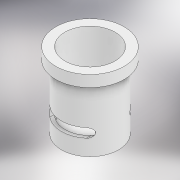
# Autodesk Inventor part: EndEffectorRotational
Saved by Autodesk Inventor 2020.3 (Build 243373000, 373)
## iProperties
Created: 2021-08-11
Part Number: EndEffectorRotational
Material: ABS Plastic
Document SubType Name: Modeling
Designer: justi
Density: 1.06 g/cm^3
Appearance: Smooth - White
Author: justi
Autodesk Inventor part; units mm, degrees
ref_plane "YZ Plane" through (0, 0, 0) normal (1, 0, 0) x (0, 1, 0)
ref_plane "XZ Plane" through (0, 0, 0) normal (0, 1, 0) x (-1, 0, 0)
ref_plane "XY Plane" through (0, 0, 0) normal (0, 0, 1) x (1, 0, 0)
sketch "Sketch1" plane through (0, 0, 0) normal (0, 1, 0) x (-1, 0, 0)
  circle A0 centre (0, 0) radius 12.5
  circle A1 centre (0, 0) radius 11
  dimension "d0" = 25
  dimension "d1" = 22
  constraints: 2 centre point, 2 coincident
  measures "d0" diameter of A0
  measures "d1" diameter of A1
extrude "Extrusion1" add sketch "Sketch1" along normal mid plane 30
sketch "Sketch2" plane through (0, 15, 0) normal (0, 1, 0) x (1, 0, 0)
  circle A0 centre (0, 0) radius 15
  circle A1 centre (0, 0) radius 12.5
  dimension "d4" = 30
  constraints: 2 centre point, 2 coincident
  measures "d4" diameter of A0
extrude "Extrusion2" add sketch "Sketch2" against normal blind 5
sketch "Sketch3" plane through (0, -15, 0) normal (0, -1, 0) x (1, 0, 0)
  circle A0 centre (0, 0) radius 12.5
  constraints: 1 centre point, 1 coincident
extrude "Extrusion3" add sketch "Sketch3" along normal blind 3
sketch "Sketch4" plane through (0, -18, 0) normal (0, -1, 0) x (1, 0, 0)
  line L0 (0, 0) -> (-5, 0)
  line L1 (0, 0) -> (5, 0)
  circle A0 centre (-5, 0) radius 2
  circle A1 centre (5, 0) radius 2
  dimension "d21" = 5
  dimension "d22" = 5
  dimension "d23" = 4
  dimension "d24" = 4
  constraints: 4 end point, 3 coincident, 2 centre point, 2 horizontal
  measures "d21" distance of L0.start L0.end
  measures "d22" distance of L0.start L1.end
  measures "d23" diameter of A0
  measures "d24" diameter of A1
extrude "Extrusion4" cut sketch "Sketch4" against normal through all
sketch "Sketch6" plane through (0, 0, 0) normal (0, 0, 1) x (1, 0, 0)
  line L0 (-12.5, 10) -> (12.5, 10) construction
  line L1 (0, 10) -> (0, 0) construction
  line L2 (0, 0) -> (0, -9) construction
  line L3 (-12.5, -18) -> (12.5, -18) construction
  line L4 (0, -9) -> (-8, -9) construction
  line L5 (-8, -9) -> (8, -9) construction
  line L6 (-8, -11) -> (8, -11)
  line L7 (8, -7) -> (-8, -7)
  arc A0 (-8, -7) -> (-8, -11) centre (-8, -9) ccw
  arc A1 (8, -11) -> (8, -7) centre (8, -9) ccw
  dimension "d14" = 10
  dimension "d15" = 9
  dimension "d16" = 8
  dimension "d17" = 16
  dimension "d18" = 4
  constraints: 14 end point, 4 point on circle, 4 tangent, 2 centre point, 2 horizontal, 2 midpoint, 1 parallel, 1 perpendicular, 1 vertical
  measures "d14" distance of L1.start L1.end
  measures "d15" distance of L1.end L2.end
  measures "d16" distance of L2.end L4.end
  measures "d17" distance of L4.end L5.end
  measures "d18" diameter of A1
extrude "Extrusion6" cut sketch "Sketch6" against normal through all both and the other way through all
equation "\"d21\" = d22"
body "Solid1"
